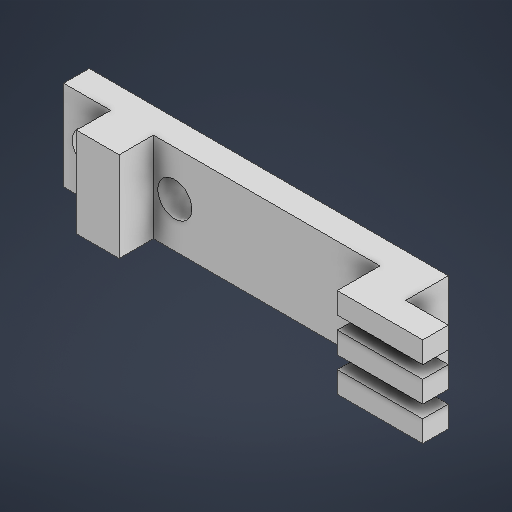
# Autodesk Inventor part: IF - TCRT5000
Saved by Autodesk Inventor 2026.2 (Build 302298010, 298A)
## iProperties
Created: 2026-03-17
Part Number: IF - TCRT5000
Material: Générique
Document SubType Name: Modeling
Designer: cleml
Density: 1 g/cm^3
Appearance: Par défaut
Author: cleml
Autodesk Inventor part; units mm, degrees
ref_plane "YZ Plane" through (0, 0, 0) normal (1, 0, 0) x (0, 1, 0)
ref_plane "XZ Plane" through (0, 0, 0) normal (0, 1, 0) x (-1, 0, 0)
ref_plane "XY Plane" through (0, 0, 0) normal (0, 0, 1) x (1, 0, 0)
sketch "Esquisse1" plane through (0, 0, 0) normal (0, 0, 1) x (1, 0, 0)
  line L0 (0, 0) -> (42, 0)
  line L1 (42, 0) -> (42, 10.5)
  line L2 (42, 10.5) -> (0, 10.5)
  line L3 (0, 10.5) -> (0, 0)
  dimension "d0" = 42
  dimension "d1" = 10.5
  constraints: 8 end point, 2 parallel, 1 horizontal, 1 perpendicular
  measures "d0" distance of L1.end L2.end
  measures "d1" distance of L0.end L1.end
extrude "Extrusion1" add sketch "Esquisse1" along normal blind 3
sketch "Esquisse2" plane through (0, 0, 3) normal (0, 0, 1) x (1, 0, 0)
  line L0 (0, 10.5) -> (0, 0) projected
  circle A0 centre (3, 5.25) radius 2
  circle A1 centre (13, 5.25) radius 2
  dimension "d4" = 3
  dimension "d5" = 10
  dimension "d6" = 4
  dimension "d7" = 4
  constraints: 2 centre point, 2 coincident
  measures "d4" distance from line of L0 point (3, 5.25)
  measures "d5" distance of point (3, 5.25) point (13, 5.25)
  measures "d6" diameter of A0
  measures "d7" diameter of A1
extrude "Extrusion2" cut sketch "Esquisse2" against normal through all
sketch "Esquisse3" plane through (0, 0, 3) normal (0, 0, 1) x (1, 0, 0)
  line L0 (0, 10.5) -> (0, 0) projected
  line L1 (0, 10.5) -> (5.5, 10.5)
  line L2 (42, 10.5) -> (0, 10.5) projected
  line L3 (5.5, 10.5) -> (10.5, 10.5)
  line L4 (10.5, 10.5) -> (10.5, 0)
  line L5 (10.5, 0) -> (5.5, 0)
  line L6 (5.5, 0) -> (5.5, 10.5)
  dimension "d10" = 5.5
  dimension "d11" = 5
  dimension "d12" = 10.5
  constraints: 10 end point, 2 parallel, 1 horizontal, 1 perpendicular, 1 point on line
  measures "d10" distance of L0.start L1.end
  measures "d11" distance of L4.end L5.end
  measures "d12" distance of L3.end L4.end
extrude "Extrusion3" add sketch "Esquisse3" along normal blind 4
sketch "Esquisse4" plane through (0, 0, 3) normal (0, 0, 1) x (1, 0, 0)
  line L0 (42, 10.5) -> (0, 10.5) projected
  line L1 (42, 10.5) -> (37, 10.5)
  line L2 (37, 10.5) -> (37, 0)
  line L3 (37, 0) -> (42, 0)
  line L4 (42, 0) -> (42, 10.5)
  point P0 (0, 0)
  dimension "d15" = 5
  dimension "d16" = 10.5
  constraints: 8 end point, 2 parallel, 1 horizontal, 1 perpendicular
  measures "d15" distance of L3.end L2.end
  measures "d16" distance of L2.end L1.end
extrude "Extrusion4" add sketch "Esquisse4" along normal blind 5
sketch "Esquisse5" plane through (42, 0, 0) normal (1, 0, 0) x (0, 0, -1)
  line L0 (-8, 10.5) -> (-8, 0) projected
  line L1 (-8, 0) -> (-5, 0)
  line L2 (-5, 0) -> (-5, 2.5)
  line L3 (-5, 2.5) -> (-8, 2.5)
  line L4 (-8, 2.5) -> (-8, 0)
  line L5 (-8, 2.5) -> (-8, 4)
  line L6 (-8, 4) -> (-5, 4)
  line L7 (-5, 4) -> (-5, 6.5)
  line L8 (-5, 6.5) -> (-8, 6.5)
  line L9 (-8, 6.5) -> (-8, 4)
  line L10 (-8, 6.5) -> (-8, 8)
  line L11 (-8, 8) -> (-5, 8)
  line L12 (-5, 8) -> (-5, 10.5)
  line L13 (-5, 10.5) -> (-8, 10.5)
  line L14 (-8, 10.5) -> (-8, 8)
  point P0 (0, 0)
  dimension "d21" = 3
  dimension "d22" = 2.5
  dimension "d23" = 1.5
  dimension "d24" = 3
  dimension "d25" = 2.5
  dimension "d26" = 1.5
  dimension "d27" = 3
  dimension "d28" = 2.5
  constraints: 28 end point, 6 parallel, 3 horizontal, 3 perpendicular, 1 point on line
  measures "d21" distance of L3.end L2.end
  measures "d22" distance of L2.end L1.end
  measures "d23" distance of L3.end L5.end
  measures "d24" distance of L8.end L7.end
  measures "d25" distance of L7.end L6.end
  measures "d26" distance of L8.end L10.end
  measures "d27" distance of L13.end L12.end
  measures "d28" distance of L12.end L11.end
extrude "Extrusion5" add sketch "Esquisse5" along normal blind 5
sketch "Esquisse6" plane through (42, 0, 0) normal (1, 0, 0) x (0, 0, -1)
  line L0 (-5, 2.5) -> (-8, 2.5) projected
  line L1 (-5, 6.5) -> (-5, 4) projected
  line L2 (-8, 2.5) -> (-5, 2.5)
  line L3 (-5, 2.5) -> (-5, 4)
  line L4 (-5, 4) -> (-8, 4)
  line L5 (-8, 4) -> (-8, 2.5)
  line L6 (-8, 6.5) -> (-5, 6.5)
  line L7 (-5, 6.5) -> (-5, 8.0213)
  line L8 (-5, 8.0213) -> (-8, 8.0213)
  line L9 (-8, 8.0213) -> (-8, 6.5)
  point P0 (0, 0)
  constraints: 16 end point, 4 parallel, 2 horizontal, 2 perpendicular, 2 point on line
extrude "Extrusion6" cut sketch "Esquisse6" against normal blind 5
